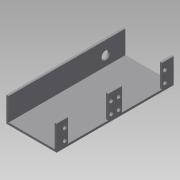
# Autodesk Inventor part: upper_leg
Saved by Autodesk Inventor 2015 (Build 190159000, 159)
## iProperties
Created: 2014-06-07
Part Number: upper_leg
Material: Generic
Document SubType Name: Modeling
Designer: L
Density: 1 g/cm^3
Appearance: Default
Mass: 130.151 g
Surface Area: 472.782 cm^2
Volume: 130.151 cm^3
Author: L
Autodesk Inventor part; units mm, degrees
ref_plane "YZ Plane" through (0, 0, 0) normal (1, 0, 0) x (0, 1, 0)
ref_plane "XZ Plane" through (0, 0, 0) normal (0, 1, 0) x (-1, 0, 0)
ref_plane "XY Plane" through (0, 0, 0) normal (0, 0, 1) x (1, 0, 0)
sketch "Sketch2" plane through (0, 0, 0) normal (0, 0, 1) x (1, 0, 0)
  line L0 (0, 0) -> (76.2, 0)
  line L1 (76.2, 0) -> (76.2, 38.1)
  line L2 (76.2, 38.1) -> (73.025, 38.1)
  line L3 (73.025, 38.1) -> (73.025, 3.175)
  line L4 (73.025, 3.175) -> (3.175, 3.175)
  line L5 (3.175, 3.175) -> (3.175, 38.1)
  line L6 (3.175, 38.1) -> (0, 38.1)
  line L7 (0, 38.1) -> (0, 0)
  dimension "d0" = 76.2
  dimension "d1" = 38.1
  dimension "d2" = 3.175
  dimension "d3" = 34.925
  dimension "d4" = 69.85
  dimension "d5" = 34.925
  dimension "d6" = 3.175
  constraints: 16 end point, 4 perpendicular, 1 horizontal, 1 point on line, 1 vertical
  measures "d0" distance of L0.start L0.end
  measures "d1" distance of L0.end L1.end
  measures "d2" distance of L1.end L2.end
  measures "d3" distance of L2.end L3.end
  measures "d4" distance of L3.end L4.end
  measures "d5" distance of L4.end L5.end
  measures "d6" distance of L5.end L6.end
extrude "Extrusion_channel" add sketch "Sketch2" along normal blind 177.8
sketch "Sketch3" plane through (76.2, 0, 0) normal (1, 0, 0) x (0, 0, -1)
  circle A0 centre (-12.7, 9.4234) radius 2.9464
  circle A1 centre (-12.7, 26.5334) radius 2.9464
  line L0 (0, 0) -> (-177.8, 0) projected
  line L1 (0, 0) -> (0, 38.1) projected
  circle A2 centre (-83.312, 9.4234) radius 2.9464
  circle A3 centre (-83.312, 26.5334) radius 2.9464
  line L2 (-78.486, 38.1) -> (-17.526, 38.1)
  line L3 (-17.526, 38.1) -> (-17.526, 3.175)
  line L4 (-17.526, 3.175) -> (-78.486, 3.175)
  line L5 (-78.486, 3.175) -> (-78.486, 38.1)
  line L6 (-78.486, 38.1) -> (-17.526, 3.175) construction
  line L7 (-17.526, 38.1) -> (-78.486, 3.175) construction
  line L8 (0, 38.1) -> (-177.8, 38.1) projected
  line L9 (-88.9, 38.1) -> (-88.9, 0)
  circle A4 centre (-165.1, 9.4234) radius 2.9464
  circle A5 centre (-165.1, 26.5334) radius 2.9464
  line L10 (-177.8, 0) -> (-177.8, 38.1)
  circle A6 centre (-94.488, 9.4234) radius 2.9464
  circle A7 centre (-94.488, 26.5334) radius 2.9464
  line L11 (-99.314, 38.1) -> (-160.274, 38.1)
  line L12 (-160.274, 38.1) -> (-160.274, 3.175)
  line L13 (-160.274, 3.175) -> (-99.314, 3.175)
  line L14 (-99.314, 3.175) -> (-99.314, 38.1)
  line L15 (-99.314, 38.1) -> (-160.274, 3.175) construction
  line L16 (-160.274, 38.1) -> (-99.314, 3.175) construction
  point P0 (-48.006, 20.6375)
  point P1 (-129.794, 20.6375)
  dimension "d9" = 5.8928
  dimension "d10" = 5.8928
  dimension "d11" = 9.4234
  dimension "d12" = 17.11
  dimension "d13" = 12.7
  dimension "d14" = 5.8928
  dimension "d15" = 5.8928
  dimension "d16" = 70.612
  dimension "d17" = 60.96
  dimension "d18" = 34.925
  dimension "d19" = 35.306
  dimension "d20" = 3.175
  constraints: 28 end point, 9 symmetric about line, 8 centre point, 6 midpoint, 2 horizontal alignment, 2 parallel, 2 vertical alignment, 1 horizontal, 1 perpendicular, 4 other
  measures "d9" diameter of A0
  measures "d10" diameter of A1
  measures "d11" distance from line of L0 A0.centre
  measures "d12" distance of A1.centre A0.centre
  measures "d13" distance from line of L1 A0.centre
  measures "d14" diameter of A2
  measures "d15" diameter of A3
  measures "d16" distance of A2.centre A0.centre
  measures "d17" distance of L3.end L4.end
  measures "d18" distance of L2.end L3.end
  measures "d19" horizontal distance of A3.centre point (-48.006, 20.638)
  measures "d20" distance between parallel lines of L0 L4
extrude "Extrusion_mount" cut sketch "Sketch3" against normal blind 3.175 contours A0 | A1 | L3 L4 L5 L2 | L14 L13 L12 L8 | A2 | A3 | A4 | A5 | A6 | A7
sketch "Sketch8" plane through (0, 0, 0) normal (-1, 0, 0) x (0, 0, 1)
  line L0 (0, 0) -> (177.8, 0) projected
  line L1 (88.9, 0) -> (169.037, 38.1)
  line L2 (160.274, 38.1) -> (177.8, 38.1) projected
  circle A0 centre (30.166, 17.9784) radius 6.35
  line L3 (0, 38.1) -> (0, 0) projected
  circle A1 centre (65.7664, -56.9012) radius 6.35
  point P0 (78.486, 38.1)
  point P1 (99.314, 38.1)
  dimension "d26" = 12.7
  dimension "d27" = 17.9784
  dimension "d28" = 30.166
  constraints: 2 centre point, 2 end point, 2 midpoint, 1 symmetric about line, 1 other
  measures "d26" diameter of A0
  measures "d27" distance from line of L0 A0.centre
  measures "d28" distance from line of L3 A0.centre
extrude "Extrusion_hole" cut sketch "Sketch8" against normal blind 3.175
equation "\"d0\" = o_width"
equation "\"d1\" = height"
equation "\"d2\" = thickness"
equation "\"d3\" = height - thickness"
equation "\"d4\" = i_width"
equation "\"d5\" = height - thickness"
equation "\"d6\" = thickness"
equation "\"d7\" = length"
equation "\"d9\" = hole_dia"
equation "\"d10\" = hole_dia"
equation "\"d11\" = hole_height"
equation "\"d12\" = hole_spacing"
equation "\"d13\" = end_space"
equation "\"d14\" = hole_dia"
equation "\"d15\" = hole_dia"
equation "\"d16\" = mount_spacing"
equation "\"d17\" = servo_space"
equation "\"d18\" = height - thickness"
equation "\"d19\" = 0.5 * mount_spacing"
equation "\"d20\" = thickness"
equation "\"d21\" = thickness"
equation "\"d26\" = mount_dia"
equation "\"d27\" = 0.5 * hole_spacing + hole_height"
equation "\"d28\" = servo_axis + end_space"
equation "\"d29\" = thickness"
equation "\"length\" = 177.8"
equation "\"o_width\" = 76.2"
equation "\"thickness\" = 3.175"
equation "\"i_width\" = o_width - 2 * thickness"
equation "\"height\" = 0.5 * o_width"
equation "\"servo_space\" = 60.96"
equation "\"mount_spacing\" = 70.612"
equation "\"hole_dia\" = 5.8928"
equation "\"end_space\" = 12.7"
equation "\"hole_spacing\" = 17.11"
equation "\"servo_axis\" = 17.466"
equation "\"mount_dia\" = 12.7"
equation "\"hole_height\" = 9.4234"
body "Solid1"
